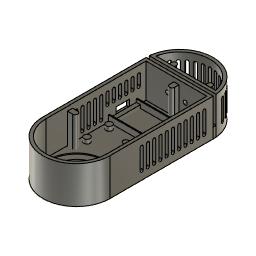
Krabicka pro termostat (Autodesk Fusion 360 design; units mm, degrees)
Autodesk Fusion 360 part; units mm, degrees
note: some values were not read from the file. Chosen so that the rebuilt part matches the saved one: which bodies a step acts on; which face or edge a step refers to. Set by a fixed rule: which sketch regions a step uses.
sketch "Sketch1" plane through (0, 0, 0) normal (0, 0, 1) x (1, 0, 0)
  circle A0 centre (0.0005, 0) radius 20.75
  arc A1 (32.4989, 100) -> (-32.5011, 100) centre (-0.0011, 100) ccw
  circle A2 centre (0.0005, 0) radius 27
  circle A3 centre (-23.4995, 33.6708) radius 3
  circle A4 centre (23.5005, 55.0015) radius 3
  circle A5 centre (23.4975, 33.1458) radius 3
  circle A6 centre (-23.4995, 55.25) radius 3
  line L0 (-26.4995, 58.5) -> (26.5005, 58.5) construction
  line L1 (26.5005, 58.5) -> (26.5005, 30) construction
  line L2 (26.5005, 30) -> (-26.4995, 30) construction
  line L3 (-26.4995, 30) -> (-26.4995, 58.5) construction
  line L4 (-49, 0) -> (63, 0)
  line L5 (-32.5011, 100) -> (32.4989, 100)
  line L6 (-32.5011, 100) -> (-32.4995, 0)
  line L7 (32.4989, 100) -> (32.5005, 0)
  arc A7 (-32.4995, 0) -> (32.5005, 0.0005) centre (0.0005, 0) ccw
  arc A8 (-29.5001, 0) -> (29.5005, 0) centre (0.0002, 0) ccw
  line L8 (-29.501, 88.5) -> (6.4991, 88.5)
  line L9 (6.4991, 88.5) -> (6.4991, 60.5)
  line L10 (6.4991, 60.5) -> (-29.5007, 60.5)
  line L11 (-29.501, 87.5) -> (5.5005, 87.5)
  line L12 (5.5005, 87.5) -> (5.5005, 61.5)
  line L13 (5.5005, 61.5) -> (-29.5007, 61.5)
  line L14 (-29.4995, 61.5) -> (-29.4995, 87.5)
  line L15 (8.7491, 92.5) -> (27.2491, 92.5) construction
  line L16 (27.2491, 92.5) -> (27.2491, 60.5) construction
  line L17 (27.2491, 60.5) -> (8.7491, 60.5) construction
  line L18 (8.7491, 60.5) -> (8.7491, 92.5) construction
  line L19 (27.2491, 74.5) -> (8.7491, 74.5)
  line L20 (27.2491, 80.5) -> (8.7491, 80.5)
  line L21 (-29.5011, 97) -> (29.4989, 97)
  line L22 (-32.3624, 103) -> (32.3601, 103)
  line L23 (-28.8845, 106) -> (28.8823, 106)
  line L24 (-6.0011, 111) -> (5.9989, 111)
  line L25 (5.9989, 111) -> (5.9989, 126)
  line L26 (5.9989, 126) -> (-6.0011, 126)
  line L27 (-6.0011, 126) -> (-6.0011, 111)
  arc A9 (-29.3482, 103) -> (-29.5011, 99.9993) centre (-0.0011, 100) ccw
  arc A10 (29.4989, 100.0007) -> (29.3459, 103) centre (-0.0011, 100) ccw
  arc A11 (28.8823, 106) -> (-28.8845, 106) centre (-0.0011, 100) ccw
  line L28 (29.4989, 100.0007) -> (29.4989, 100)
  line L29 (29.4989, 97) -> (29.5005, 0)
  line L30 (-29.5011, 97) -> (-29.5001, 0)
  line L31 (8.7491, 80.5) -> (8.7491, 74.5)
  line L32 (27.2491, 80.5) -> (27.2491, 74.5)
  line L33 (-24.4995, 23.2909) -> (-38.4097, 23.2907) construction
  line L34 (-24.4995, 20.7909) -> (-29.5003, 20.7908)
  line L35 (-24.4996, 25.7909) -> (-29.5003, 25.7908)
  arc A12 (-24.4995, 20.7909) -> (-24.4996, 25.7909) centre (-24.4995, 23.2909) ccw
  line L36 (24.4992, 20.7913) -> (29.5001, 20.7913)
  arc A13 (24.4992, 25.7913) -> (24.4992, 20.7913) centre (24.4992, 23.2913) ccw
  line L37 (24.4992, 25.7913) -> (29.5001, 25.7913)
  line L38 (-29.5011, 97) -> (-29.5001, 0)
  line L39 (-2.5011, 92.75) -> (-2.5011, 97)
  line L40 (2.4989, 92.75) -> (2.4989, 97)
  arc A14 (-2.5011, 92.75) -> (2.4989, 92.75) centre (-0.0011, 92.75) ccw
  line L41 (-26.4995, 112) -> (22.6043, 112) construction
  line L42 (-20.0011, 112) -> (-20.0011, 106)
  line L43 (-15.0011, 112) -> (-15.0011, 106)
  arc A15 (-15.0011, 112) -> (-20.0011, 112) centre (-17.5011, 112) ccw
  line L44 (14.9994, 112) -> (15, 106)
  line L45 (19.9994, 112) -> (19.9994, 106)
  arc A16 (19.9994, 112) -> (14.9994, 112) centre (17.4994, 112.0003) ccw
  line L46 (0.0002, 0) -> (0.0007, -38) construction
  line L47 (-1.7495, -20.75) -> (1.7505, -20.75)
  line L48 (-1.7495, -22.75) -> (1.7505, -22.75)
  line L49 (-1.7495, -20.75) -> (-1.7495, -22.75)
  line L50 (1.7505, -20.75) -> (1.7505, -22.75)
  line L51 (20.7505, 1.75) -> (22.7505, 1.75)
  line L52 (20.7505, -1.75) -> (22.7505, -1.75)
  line L53 (20.7505, -1.75) -> (20.7505, 1.75)
  line L54 (22.7505, -1.75) -> (22.7505, 1.75)
  line L55 (-1.7495, 20.75) -> (-1.7496, 22.75)
  line L56 (1.7505, 20.75) -> (1.7504, 22.75)
  line L57 (1.7505, 20.75) -> (-1.7495, 20.75)
  line L58 (1.7505, 22.75) -> (-1.7496, 22.75)
  line L59 (-20.7495, -1.75) -> (-22.7495, -1.75)
  line L60 (-20.7495, 1.75) -> (-22.7495, 1.75)
  line L61 (-20.7495, 1.75) -> (-20.7495, -1.75)
  line L62 (-22.7495, 1.75) -> (-22.7495, -1.75)
  line L63 (5.5005, 74.5) -> (-60, 74.5) construction
  line L64 (-25.4995, 61.5) -> (-25.4995, 87.5)
  line L65 (1.5005, 87.5) -> (1.5005, 61.5)
  dimension "d2" = 41.5
  dimension "d3" = 65
  dimension "d65" = 6
  dimension "d66" = 6
  dimension "d68" = 6
  dimension "d69" = 6
  dimension "d70" = 47
  dimension "d72" = 47
  dimension "d76" = 54
  dimension "d79" = 53
  dimension "d80" = 28.5
  dimension "d82" = 3.25
  dimension "d88" = 65
  dimension "d91" = 100
  dimension "d92" = 6
  dimension "d93" = 9
  dimension "d94" = 9
  dimension "d99" = 30
  dimension "d104" = 28
  dimension "d107" = 3
  dimension "d109" = 18.5
  dimension "d110" = 32
  dimension "d111" = 2
  dimension "d112" = 2.25
  dimension "d114" = 35
  dimension "d115" = 14
  dimension "d116" = 6
  dimension "d118" = 26
  dimension "d122" = 12
  dimension "d123" = 15
  dimension "d124" = 6
  dimension "d125" = 5
  dimension "d144" = 5
  dimension "d145" = 8
  dimension "d148" = 5
  dimension "d149" = 4.25
  dimension "d150" = 32.5
  dimension "d151" = 5
  dimension "d152" = 15
  dimension "d153" = 12
  dimension "d226" = 360
  dimension "d229" = 4
  constraint horizontal L0
  constraint vertical L1
  constraint horizontal L2
  constraint vertical L3
  constraint concentric A0 A2
  constraint horizontal L4
  constraint concentric A0 A7
  constraint coincident L4 L6.end
  constraint coincident L7.end A7
  constraint coincident L4 L7.end
  constraint coincident L7 A7.end
  constraint coincident L4 A8.start
  constraint horizontal L8
  constraint vertical L9
  constraint horizontal L10
  constraint parallel L8 L11
  constraint parallel L9 L12
  constraint parallel L10 L13
  constraint horizontal L15
  constraint vertical L16
  constraint horizontal L17
  constraint vertical L18
  constraint horizontal L19
  constraint horizontal L20
  constraint horizontal L24
  constraint vertical L25
  constraint horizontal L26
  constraint vertical L27
  constraint parallel L5 L23
  constraint concentric A1 A10
  constraint parallel L7 L28
  constraint coincident L22 A9.start
  constraint concentric A9 A10
  constraint coincident L22 A10.end
  constraint concentric A10 A11
  constraint parallel L5 L22
  constraint coincident A1 L22.end
  constraint coincident A1 L22.start
  constraint parallel L5 L21
  constraint coincident L21.end L28
  constraint coincident L5 L28.end
  constraint collinear L28 L29
  constraint coincident L30 L11.start
  constraint coincident L14.end L11
  constraint coincident L30 L13.end
  constraint coincident L14.start L13
  constraint coincident L30 L8.start
  constraint coincident L30 L10.end
  constraint perpendicular L19 L31
  constraint perpendicular L19 L32
  constraint coincident L33.start A12.centre
  constraint parallel L33 L34
  constraint coincident L30 L34.end
  constraint parallel L33 L35
  constraint coincident L30 L35.end
  constraint coincident L39.start A14
  constraint perpendicular L21 L39
  constraint perpendicular L21 L40
  constraint coincident L39 A14.start
  constraint coincident L21 L39.end
  constraint coincident L21 L40.end
  constraint perpendicular L27 L41
  constraint coincident L41 L42.start
  constraint tangent L42 A15
  constraint perpendicular L23 L42
  constraint coincident L41 L43.start
  constraint tangent L43 A15
  constraint perpendicular L23 L43
  constraint coincident L23 L42.end
  constraint coincident L23 L43.end
  constraint coincident L41 L44.start
  constraint tangent L44 A16
  constraint coincident L41 L45.start
  constraint perpendicular L23 L45
  constraint coincident L23 L45.end
  constraint coincident L23 L44.end
  constraint coincident A8.centre L46.start
  constraint tangent A0 L47
  constraint horizontal L47
  constraint parallel L47 L48
  constraint parallel L46 L50
  constraint coincident L48 L49.end
  constraint midpoint L12 L63.start
  constraint perpendicular L12 L63
  constraint parallel L12 L65
  constraint coincident L11 L65.start
  constraint coincident L13 L65.end
  measures "d2" diameter of A0
  measures "d3" diameter of A1
  measures "d65" diameter of A3
  measures "d66" diameter of A4
  measures "d68" diameter of A5
  measures "d69" diameter of A6
  measures "d70" distance of A3.centre A5.centre
  measures "d72" horizontal distance of A4.centre A6.centre
  measures "d76" diameter of A2
  measures "d79" distance of L0.start L0.end
  measures "d80" distance of L0.start L2.end
  measures "d82" vertical distance of A6.centre L0.start
  measures "d88" diameter of A7
  measures "d91" vertical distance of A1.centre A0.centre
  measures "d92" horizontal distance of L2.end L6.end
  measures "d93" horizontal distance of A3.centre L6.end
  measures "d94" horizontal distance of A6.centre L6.end
  measures "d99" vertical distance of L2.end L4.start
  measures "d104" distance of L8.end L9.end
  measures "d107" horizontal distance of L6.end L14.start
  measures "d109" distance of L15.start L15.end
  measures "d110" distance of L15.start L17.end
  measures "d111" vertical distance of L0.start L17.end
  measures "d112" distance of L9.end L17.end
  measures "d114" distance of L14.end L11.end
  measures "d115" distance of L16.end L19.start
  measures "d116" distance of L19.start L20.start
  measures "d118" distance of L14.end L14.start
  measures "d122" distance of L24.start L24.end
  measures "d123" distance of L24.start L26.end
  measures "d124" horizontal distance of A1.centre L24.end
  measures "d125" vertical distance of L24.end L23.end
  measures "d144" diameter of A12
  measures "d145" horizontal distance of L6.end L33.start
  measures "d148" diameter of A14
  measures "d149" vertical distance of L21.start A14.centre
  measures "d150" horizontal distance of A1.end A14.centre
  measures "d151" diameter of A15
  measures "d152" horizontal distance of A1.end A15.centre
  measures "d153" vertical distance of A1.end A15.centre
extrude "Extrude11" add sketch "Sketch1" along normal blind 2 contours L47 L48 L49 L50 | A0 A2 L4 L52 L53 L54 L59 L61 L62 | L4 L51 L53 L54 | L4 L52 L53 L54 | L55 L56 L57 L58 | A0 A2 L4 L51 L53 L54 L60 L61 L62 | L4 L59 L61 L62 | L4 L60 L61 L62 makes body 1
extrude "Extrude12" add sketch "Sketch1" along normal blind 3 separate body contours A2 L4 A8 | A2 L4 L8 L9 L10 L21 L29 L30 L34 L35 A12 L36 A13 L37 L38 L39 L40 A14 | L29 L36 A13 L37 | L30 L34 L35 A12 L38 | L5 L22 A9 A10 | L21 L39 L40 A14 | L11 L13 L14 L30 L38 L64 | L11 L13 L64 L65 | L11 L12 L13 L65 | L19 L20 L31 L32 | L23 A11 L42 L43 A15 L44 L45 A16 | L23 L42 L43 A15 | L23 L44 L45 A16 makes body 2 at (-9.8345, 100, 1) makes body 3 at (-5.4383, 47.1243, 0) makes body 4 at (8.7413, 120.9475, 0) makes body 5 at (-17.8337, 78.8333, 0)
extrude "Extrude13" add sketch "Sketch1" along normal blind 36 separate body contours L4 L5 L6 L7 L14 L21 L29 L30 L38 | L4 A7 A8 | A1 L22 makes body 6 at (21.5052, -24.3679, 24) makes body 7 at (-32.1753, 104.5904, 24)
extrude "Extrude14" add sketch "Sketch1" along normal blind 10 separate body contours A1 L5 L22 A10 | A1 L5 L22 A9 makes body 8 at (30.3507, 103, 3.3333) makes body 9 at (-31.3576, 103, 3.3333)
extrude "Extrude15" add sketch "Sketch1" along normal blind 7 separate body contours A3 | A4 | A5 | A6 makes body 10 at (-26.4846, 54.9513, 4.6667) makes body 11 at (20.5154, 54.7028, 4.6667) makes body 12 at (-26.4846, 33.3721, 4.6667) makes body 13 at (20.5124, 32.8471, 4.6667)
extrude "Extrude16" add sketch "Sketch1" along normal blind 9 separate body contours L8 L9 L10 L11 L12 L13 L30 L38 makes body 14
extrude "Extrude17" add sketch "Sketch1" along normal blind 8 separate body contours L24 L25 L26 L27 makes body 15
extrude "Extrude18" add sketch "Sketch1" along normal blind 7 separate body contours L19 L20 L31 L32 makes body 16
extrude "Extrude19" add sketch "Sketch1" along normal blind 32 separate body contours L29 L36 A13 L37 | L30 L34 L35 A12 L38 | L21 L39 L40 A14 | L23 L42 L43 A15 | L23 L44 L45 A16 makes body 17 at (19.9221, 112.6169, 21.3333) makes body 18 at (22.3991, 24.6477, 21.3333) makes body 19 at (-19.6343, 113.3036, 10.6667) makes body 20 at (-22.8925, 21.3758, 21.3333) makes body 21 at (2.4216, 92.1331, 21.3333)
sketch "Sketch6" plane through (0, 100, 0) normal (0, 1, 0) x (-1, 0, 0)
  line L0 (-32.4989, 0) -> (32.5011, 0)
  line L1 (32.5011, 0) -> (32.5011, 36)
  line L2 (32.5011, 36) -> (-32.4989, 36)
  line L3 (-32.4989, 36) -> (-32.4989, 0)
  line L4 (0, 0) -> (0, 60.6352)
  line L5 (-45, 18) -> (-11, 18) construction
  line L6 (0, 40) -> (0, 4) construction
  line L7 (-1.5, 18) -> (-1.5, 8)
  line L8 (1.5, 18) -> (1.5, 8)
  arc A0 (-1.5, 8) -> (1.5, 8) centre (0, 8) ccw
  arc A1 (1.5, 28) -> (-1.5, 28) centre (0, 28) ccw
  line L9 (1.5, 18) -> (1.5, 28)
  line L10 (-1.5, 18) -> (-1.5, 28)
  line L11 (32.5011, 36) -> (-32.4989, 36)
  line L12 (-32.4989, 36) -> (-32.4989, 0)
  line L13 (-32.4989, 0) -> (32.5011, 0)
  line L14 (32.5011, 0) -> (32.5011, 36)
  circle A2 centre (8.5011, 20) radius 2
  circle A3 centre (8.5011, 20) radius 3
  circle A4 centre (-8.5011, 20) radius 3
  circle A5 centre (-8.5011, 20) radius 2
  point P0 (-63, 0)
  dimension "d167" = 3
  dimension "d170" = 10
  dimension "d171" = 8
  dimension "d172" = 1.5
  dimension "d188" = 4
  dimension "d189" = 6
  dimension "d190" = 20
  dimension "d191" = 24
  constraint coincident L4.start origin
  constraint vertical L4
  constraint horizontal L5
  constraint vertical L6
  constraint coincident A0.centre L6
  constraint parallel L6 L7
  constraint parallel L6 L8
  constraint coincident L5 L7.start
  constraint coincident L5 L8.start
  constraint symmetric L5 L7.end A1.end
  constraint symmetric L5 L8.end A1.start
  constraint symmetric L5 A0 A1
  constraint symmetric L5 L7.start L10.start
  constraint symmetric L5 L8.start L9.start
  constraint horizontal L11
  constraint vertical L12
  constraint horizontal L13
  constraint vertical L14
  constraint coincident L0.start L3.end
  constraint coincident L1.end L2.start
  constraint concentric A2 A3
  constraint symmetric L4 A2 A5
  constraint symmetric L4 A3 A4
  measures "d167" diameter of A0
  measures "d170" vertical distance of A0.centre L5.start
  measures "d171" vertical distance of A0.centre P0
  measures "d172" distance of L4 L7.end
  measures "d188" diameter of A2
  measures "d189" diameter of A3
  measures "d190" vertical distance of L0.end A2.centre
  measures "d191" distance of L14 A2.centre
extrude "Extrude21" add sketch "Sketch6" along normal blind 68 separate body contours L4 L7 A0 A1 L10 | L4 L8 A0 A1 L9 makes body 22
pattern_circular "C-Pattern1" count 7 over 70 about axis through (0, 100, 0) along (0, 0, 1) of bodies 22 makes body 23 at (-7.6982, 144.7001, 21.3333) makes body 24 at (-7.6005, 121.407, 21.3333) makes body 25 at (-11.7723, 119.4278, 21.3333) makes body 26 at (-31.9449, 132.2007, 24.6667) makes body 27 at (-37.7965, 125.0756, 21.3333) makes body 28 at (-42.0864, 116.9145, 21.3333)
pattern_circular "C-Pattern2" count 7 over 70 about axis through (0, 100, 0) along (0, 0, -1) of bodies 22 makes body 29 at (10.6362, 144.0934, 21.3333) makes body 30 at (19.3329, 141.0317, 21.3333) makes body 31 at (14.2298, 117.7071, 21.3333) makes body 32 at (17.5165, 114.4638, 24.6667) makes body 33 at (39.3714, 122.5223, 21.3333) makes body 34 at (43.1124, 114.0954, 24.6667)
extrude "Extrude22" add sketch "Sketch6" along normal blind 7 separate body contours L0 L2 L3 L4 L7 A0 A1 L10 L11 L12 L13 | L0 L1 L2 L4 L8 A0 A1 L9 L11 L13 L14 | L4 L7 A0 A1 L10 | L4 L8 A0 A1 L9 | A2 | A3 | A4 | A5 makes body 35
combine "Combine1" operation cut target body 28 tool bodies 35 keep tools makes body 36 at (-1.4619, 100, 14.6667)
combine "Combine2" operation cut target body 27 tool bodies 35 keep tools makes body 37 at (-0.9524, 100, 14.6667)
combine "Combine3" operation cut target body 26 tool bodies 35 keep tools makes body 38 at (-0.7286, 100, 21.3333)
combine "Combine4" operation cut target body 25 tool bodies 35 keep tools makes body 39 at (-0.6104, 100, 21.3333)
combine "Combine5" operation cut target body 24 tool bodies 35 keep tools makes body 40 at (-0.5445, 100, 14.6667)
combine "Combine6" operation cut target body 23 tool bodies 35 keep tools makes body 41 at (-0.5105, 100, 14.6667)
combine "Combine7" operation cut target body 22 tool bodies 35 keep tools
combine "Combine8" operation cut target body 29 tool bodies 35 keep tools makes body 42 at (0.5105, 100, 21.3333)
combine "Combine9" operation cut target body 30 tool bodies 35 keep tools makes body 43 at (0.5445, 100, 21.3333)
combine "Combine10" operation cut target body 31 tool bodies 35 keep tools makes body 44 at (0.6104, 100, 21.3333)
combine "Combine11" operation cut target body 32 tool bodies 35 keep tools makes body 45 at (0.7286, 100, 21.3333)
combine "Combine12" operation cut target body 33 tool bodies 35 keep tools makes body 46 at (0.9524, 100, 21.3333)
combine "Combine13" operation cut target body 34 tool bodies 35 makes body 47 at (1.4619, 100, 21.3333)
combine "Combine14" operation cut target body 7 tool bodies 28 27 26 25 24 23 22 29 30 31 32 33 34
combine "Combine15" operation add target body 6 tool bodies 36 37 38 39 40 41 42 43 44 45 46 47
sketch "Sketch8" plane through (6.4991, 0, 0) normal (1, 0, 0) x (0, 1, 0)
  line L0 (60.5, 0) -> (88.5, 0)
  line L1 (88.5, 0) -> (88.5, 9)
  line L2 (88.5, 9) -> (60.5, 9)
  line L3 (60.5, 9) -> (60.5, 0)
  line L4 (68, 12) -> (81, 12)
  line L5 (81, 12) -> (81, 5)
  line L6 (81, 5) -> (68, 5)
  line L7 (68, 5) -> (68, 12)
  line L8 (0, 3) -> (97, 3)
  dimension "d181" = 13
  dimension "d182" = 7
  dimension "d183" = 5
  dimension "d184" = 7.5
  constraint horizontal L4
  constraint vertical L5
  constraint horizontal L6
  constraint vertical L7
  measures "d181" distance of L5.end L6.end
  measures "d182" distance of L4.end L5.end
  measures "d183" vertical distance of L0.start L6.end
  measures "d184" distance of L3 L6.end
extrude "Extrude23" add sketch "Sketch8" against normal blind 43 separate body contours L2 L4 L5 L7 | L2 L5 L6 L7 makes body 48
combine "Combine16" operation cut target body 6 tool bodies 48
extrude "Extrude24" add sketch "Sketch6" along normal blind 6 separate body contours A4 makes body 49
extrude "Extrude25" add sketch "Sketch6" along normal blind 6 separate body contours A3 makes body 50
extrude "Extrude26" add sketch "Sketch6" along normal mid plane 20 separate body contours A2 | A5 makes body 51 at (-10.4986, 106.6667, 19.9003) makes body 52 at (6.5036, 106.6667, 19.9003)
combine "Combine17" operation cut target body 6 tool bodies 51 52 keep tools
combine "Combine18" operation cut target body 7 tool bodies 51 52
sketch "Sketch10" plane through (32.5005, 0.0005, 0) normal (1, 0.000016, 0) x (-0.000016, 1, 0)
  line L0 (0, 0) -> (99.9995, 0)
  line L1 (99.9995, 0) -> (99.9995, 36)
  line L2 (99.9995, 36) -> (0, 36)
  line L3 (-13.5, 18) -> (31.5, 18) construction
  line L4 (6.5, 8) -> (6.5, 78) construction
  line L5 (32.2857, 8) -> (32.2857, 18)
  line L6 (29.2857, 8) -> (29.2857, 18)
  line L7 (29.2857, 28) -> (29.2857, 18)
  line L8 (32.2857, 28) -> (32.2857, 18)
  arc A0 (32.2857, 28) -> (29.2857, 28) centre (30.7857, 28) ccw
  arc A1 (29.2857, 8) -> (32.2857, 8) centre (30.7857, 8) ccw
  line L9 (38.3571, 8) -> (38.3571, 18)
  line L10 (35.3571, 8) -> (35.3571, 18)
  line L11 (35.3571, 28) -> (35.3571, 18)
  line L12 (38.3571, 28) -> (38.3571, 18)
  arc A2 (38.3571, 28) -> (35.3571, 28) centre (36.8571, 28) ccw
  arc A3 (35.3571, 8) -> (38.3571, 8) centre (36.8571, 8) ccw
  line L13 (44.4286, 8) -> (44.4286, 18)
  line L14 (41.4286, 8) -> (41.4286, 18)
  line L15 (41.4286, 28) -> (41.4286, 18)
  line L16 (44.4286, 28) -> (44.4286, 18)
  arc A4 (44.4286, 28) -> (41.4286, 28) centre (42.9286, 28) ccw
  arc A5 (41.4286, 8) -> (44.4286, 8) centre (42.9286, 8) ccw
  line L17 (50.5, 8) -> (50.5, 18)
  line L18 (47.5, 8) -> (47.5, 18)
  line L19 (47.5, 28) -> (47.5, 18)
  line L20 (50.5, 28) -> (50.5, 18)
  arc A6 (50.5, 28) -> (47.5, 28) centre (49, 28) ccw
  arc A7 (47.5, 8) -> (50.5, 8) centre (49, 8) ccw
  line L21 (56.5714, 8) -> (56.5714, 18)
  line L22 (53.5714, 8) -> (53.5714, 18)
  line L23 (53.5714, 28) -> (53.5714, 18)
  line L24 (56.5714, 28) -> (56.5714, 18)
  arc A8 (56.5714, 28) -> (53.5714, 28) centre (55.0714, 28) ccw
  arc A9 (53.5714, 8) -> (56.5714, 8) centre (55.0714, 8) ccw
  line L25 (62.6429, 8) -> (62.6429, 18)
  line L26 (59.6429, 8) -> (59.6429, 18)
  line L27 (59.6429, 28) -> (59.6429, 18)
  line L28 (62.6429, 28) -> (62.6429, 18)
  arc A10 (62.6429, 28) -> (59.6429, 28) centre (61.1429, 28) ccw
  arc A11 (59.6429, 8) -> (62.6429, 8) centre (61.1429, 8) ccw
  line L29 (68.7143, 8) -> (68.7143, 18)
  line L30 (65.7143, 8) -> (65.7143, 18)
  line L31 (65.7143, 28) -> (65.7143, 18)
  line L32 (68.7143, 28) -> (68.7143, 18)
  arc A12 (68.7143, 28) -> (65.7143, 28) centre (67.2143, 28) ccw
  arc A13 (65.7143, 8) -> (68.7143, 8) centre (67.2143, 8) ccw
  line L33 (74.7857, 8) -> (74.7857, 18)
  line L34 (71.7857, 8) -> (71.7857, 18)
  line L35 (71.7857, 28) -> (71.7857, 18)
  line L36 (74.7857, 28) -> (74.7857, 18)
  arc A14 (74.7857, 28) -> (71.7857, 28) centre (73.2857, 28) ccw
  arc A15 (71.7857, 8) -> (74.7857, 8) centre (73.2857, 8) ccw
  line L37 (80.8571, 8) -> (80.8571, 18)
  line L38 (77.8571, 8) -> (77.8571, 18)
  line L39 (77.8571, 28) -> (77.8571, 18)
  line L40 (80.8571, 28) -> (80.8571, 18)
  arc A16 (80.8571, 28) -> (77.8571, 28) centre (79.3571, 28) ccw
  arc A17 (77.8571, 8) -> (80.8571, 8) centre (79.3571, 8) ccw
  line L41 (86.9286, 8) -> (86.9286, 18)
  line L42 (83.9286, 8) -> (83.9286, 18)
  line L43 (83.9286, 28) -> (83.9286, 18)
  line L44 (86.9286, 28) -> (86.9286, 18)
  arc A18 (86.9286, 28) -> (83.9286, 28) centre (85.4286, 28) ccw
  arc A19 (83.9286, 8) -> (86.9286, 8) centre (85.4286, 8) ccw
  line L45 (93, 8) -> (93, 18)
  line L46 (90, 8) -> (90, 18)
  line L47 (90, 28) -> (90, 18)
  line L48 (93, 28) -> (93, 18)
  arc A20 (93, 28) -> (90, 28) centre (91.5, 28) ccw
  arc A21 (90, 8) -> (93, 8) centre (91.5, 8) ccw
  dimension "d199" = 10
  dimension "d203" = 18
  constraint horizontal L3
  measures "d199" vertical distance of L3.start L4.start
  measures "d203" vertical distance of L2.end L3.start
sketch "Sketch11" plane through (-32.4995, -0.0005, 0) normal (-1, -0.000016, 0) x (0.000016, -1, 0)
  line L0 (-81.0005, 5) -> (-81.0005, 12)
  line L1 (-81.0005, 12) -> (-68.0005, 12)
  line L2 (-68.0005, 12) -> (-68.0005, 5)
  line L3 (-68.0005, 5) -> (-81.0005, 5)
  line L4 (-100.0005, 0) -> (-0.0005, 0)
  line L5 (-0.0005, 0) -> (-0.0005, 36)
  line L6 (-0.0005, 36) -> (-100.0005, 36)
  line L7 (-100.0005, 36) -> (-100.0005, 0)
  line L8 (-22, 18) -> (11, 18) construction
  line L9 (-29.2857, 31) -> (-29.2857, 5) construction
  line L10 (-35.3571, 31) -> (-35.3571, 5) construction
  line L11 (-41.4286, 31) -> (-41.4286, 5) construction
  line L12 (-47.5, 31) -> (-47.5, 5) construction
  line L13 (-53.5714, 31) -> (-53.5714, 5) construction
  line L14 (-59.6429, 31) -> (-59.6429, 5) construction
  line L15 (-65.7143, 31) -> (-65.7143, 5) construction
  line L16 (-71.7857, 31) -> (-71.7857, 5) construction
  line L17 (-77.8571, 31) -> (-77.8571, 5) construction
  line L18 (-83.9286, 31) -> (-83.9286, 5) construction
  line L19 (-90, 31) -> (-90, 5) construction
  arc A0 (-30.7857, 8) -> (-27.7857, 8) centre (-29.2857, 8) ccw
  line L20 (-27.7857, 18) -> (-27.7857, 8)
  line L21 (-30.7857, 18) -> (-30.7857, 8)
  line L22 (-30.7857, 18) -> (-30.7857, 28)
  arc A1 (-27.7857, 28) -> (-30.7857, 28) centre (-29.2857, 28) ccw
  line L23 (-27.7857, 18) -> (-27.7857, 28)
  arc A2 (-36.8571, 8) -> (-33.8571, 8) centre (-35.3571, 8) ccw
  line L24 (-33.8571, 18) -> (-33.8571, 8)
  line L25 (-36.8571, 18) -> (-36.8571, 8)
  line L26 (-36.8571, 18) -> (-36.8571, 28)
  arc A3 (-33.8571, 28) -> (-36.8571, 28) centre (-35.3571, 28) ccw
  line L27 (-33.8571, 18) -> (-33.8571, 28)
  arc A4 (-42.9286, 8) -> (-39.9286, 8) centre (-41.4286, 8) ccw
  line L28 (-39.9286, 18) -> (-39.9286, 8)
  line L29 (-42.9286, 18) -> (-42.9286, 8)
  line L30 (-42.9286, 18) -> (-42.9286, 28)
  arc A5 (-39.9286, 28) -> (-42.9286, 28) centre (-41.4286, 28) ccw
  line L31 (-39.9286, 18) -> (-39.9286, 28)
  arc A6 (-49, 8) -> (-46, 8) centre (-47.5, 8) ccw
  line L32 (-46, 18) -> (-46, 8)
  line L33 (-49, 18) -> (-49, 8)
  line L34 (-49, 18) -> (-49, 28)
  arc A7 (-46, 28) -> (-49, 28) centre (-47.5, 28) ccw
  line L35 (-46, 18) -> (-46, 28)
  arc A8 (-55.0714, 8) -> (-52.0714, 8) centre (-53.5714, 8) ccw
  line L36 (-52.0714, 18) -> (-52.0714, 8)
  line L37 (-55.0714, 18) -> (-55.0714, 8)
  line L38 (-55.0714, 18) -> (-55.0714, 28)
  arc A9 (-52.0714, 28) -> (-55.0714, 28) centre (-53.5714, 28) ccw
  line L39 (-52.0714, 18) -> (-52.0714, 28)
  line L40 (-61.1429, 18) -> (-61.1429, 28)
  arc A10 (-58.1429, 28) -> (-61.1429, 28) centre (-59.6429, 28) ccw
  line L41 (-58.1429, 18) -> (-58.1429, 28)
  arc A11 (-61.1429, 18) -> (-58.1429, 18) centre (-59.6429, 18) ccw
  arc A12 (-64.2143, 28) -> (-67.2143, 28) centre (-65.7143, 28) ccw
  line L42 (-64.2143, 18) -> (-64.2143, 28)
  arc A13 (-67.2143, 18) -> (-64.2143, 18) centre (-65.7143, 18) ccw
  line L43 (-67.2143, 18) -> (-67.2143, 28)
  arc A14 (-70.2857, 28) -> (-73.2857, 28) centre (-71.7857, 28) ccw
  line L44 (-70.2857, 18) -> (-70.2857, 28)
  arc A15 (-73.2857, 18) -> (-70.2857, 18) centre (-71.7857, 18) ccw
  line L45 (-73.2857, 18) -> (-73.2857, 28)
  line L46 (-76.3571, 18) -> (-76.3571, 28)
  arc A16 (-76.3571, 28) -> (-79.3571, 28) centre (-77.8571, 28) ccw
  line L47 (-79.3571, 18) -> (-79.3571, 28)
  arc A17 (-79.3571, 18) -> (-76.3571, 18) centre (-77.8571, 18) ccw
  arc A18 (-82.4286, 28) -> (-85.4286, 28) centre (-83.9286, 28) ccw
  line L48 (-85.4286, 18) -> (-85.4286, 28)
  arc A19 (-85.4286, 18) -> (-82.4286, 18) centre (-83.9286, 18) ccw
  line L49 (-82.4286, 18) -> (-82.4286, 28)
  arc A20 (-88.5, 28) -> (-91.5, 28) centre (-90, 28) ccw
  line L50 (-88.5, 18) -> (-88.5, 28)
  arc A21 (-91.5, 18) -> (-88.5, 18) centre (-90, 18) ccw
  line L51 (-91.5, 18) -> (-91.5, 28)
  dimension "d213" = 18
  constraint midpoint L14 A11.centre
  constraint tangent L41 A11
  constraint tangent L42 A13
  constraint tangent L44 A15
  constraint tangent L46 A17
  constraint tangent A19 L49
  constraint tangent L50 A21
  measures "d213" vertical distance of origin L8.end
extrude "Extrude27" add sketch "Sketch1" along normal blind 4 separate body contours L47 L48 L49 L50 | L4 L51 L53 L54 | L4 L52 L53 L54 | L55 L56 L57 L58 | L4 L59 L61 L62 | L4 L60 L61 L62 makes body 53 at (0.5838, 22.75, 1.3333) makes body 54 at (22.7505, -0.5833, 1.3333) makes body 55 at (-22.7495, 0.5833, 1.3333) makes body 56 at (-0.5829, -22.75, 1.3333)
extrude "Extrude28" add sketch "Sketch1" along normal blind 6 separate body contours L11 L13 L14 L30 L38 L64 makes body 57
extrude "Extrude29" add sketch "Sketch1" along normal blind 5 separate body contours L11 L12 L13 L65 makes body 58
extrude "Extrude30" cut sketch "Sketch10" against normal blind 3 bodies 6
extrude "Extrude31" cut sketch "Sketch11" against normal blind 3 contours A0 L20 L21 L22 A1 L23 | A2 L24 L25 L26 A3 L27 | A4 L28 L29 L30 A5 L31 | A6 L32 L33 L34 A7 L35 | A8 L36 L37 L38 A9 L39 | L40 A10 L41 A11 | A12 L42 A13 L43 | A14 L44 A15 L45 | L46 A16 L47 A17 | A18 L48 A19 L49 | A20 L50 A21 L51 bodies 6
extrude "Extrude6" [suppressed]
extrude "Extrude7" [suppressed]
sketch "Sketch3" plane through (-30, 0, 0) normal (-1, 0, 0) x (0, -1, 0)
  line L0 (-60, 0) -> (0, 0)
  line L1 (0, 0) -> (0, 36)
  line L2 (0, 36) -> (-60, 36)
  line L3 (-60, 36) -> (-60, 0)
  line L4 (-52, 8) -> (-52, 28)
  line L5 (-55, 28) -> (-55, 8)
  arc A0 (-52, 28) -> (-55, 28) centre (-53.5, 28) ccw
  arc A1 (-55, 8) -> (-52, 8) centre (-53.5, 8) ccw
  arc A2 (-46.125, 28) -> (-49.125, 28) centre (-47.625, 28) ccw
  line L6 (-46.125, 8) -> (-46.125, 28)
  line L7 (-49.125, 28) -> (-49.125, 8)
  arc A3 (-49.125, 8) -> (-46.125, 8) centre (-47.625, 8) ccw
  arc A4 (-40.25, 28) -> (-43.25, 28) centre (-41.75, 28) ccw
  line L8 (-40.25, 8) -> (-40.25, 28)
  line L9 (-43.25, 28) -> (-43.25, 8)
  arc A5 (-43.25, 8) -> (-40.25, 8) centre (-41.75, 8) ccw
  arc A6 (-34.375, 28) -> (-37.375, 28) centre (-35.875, 28) ccw
  line L10 (-34.375, 8) -> (-34.375, 28)
  line L11 (-37.375, 28) -> (-37.375, 8)
  arc A7 (-37.375, 8) -> (-34.375, 8) centre (-35.875, 8) ccw
  arc A8 (-28.5, 28) -> (-31.5, 28) centre (-30, 28) ccw
  line L12 (-28.5, 8) -> (-28.5, 28)
  line L13 (-31.5, 28) -> (-31.5, 8)
  arc A9 (-31.5, 8) -> (-28.5, 8) centre (-30, 8) ccw
  arc A10 (-22.625, 28) -> (-25.625, 28) centre (-24.125, 28) ccw
  line L14 (-22.625, 8) -> (-22.625, 28)
  line L15 (-25.625, 28) -> (-25.625, 8)
  arc A11 (-25.625, 8) -> (-22.625, 8) centre (-24.125, 8) ccw
  arc A12 (-16.75, 28) -> (-19.75, 28) centre (-18.25, 28) ccw
  line L16 (-16.75, 8) -> (-16.75, 28)
  line L17 (-19.75, 28) -> (-19.75, 8)
  arc A13 (-19.75, 8) -> (-16.75, 8) centre (-18.25, 8) ccw
  arc A14 (-10.875, 28) -> (-13.875, 28) centre (-12.375, 28) ccw
  line L18 (-10.875, 8) -> (-10.875, 28)
  line L19 (-13.875, 28) -> (-13.875, 8)
  arc A15 (-13.875, 8) -> (-10.875, 8) centre (-12.375, 8) ccw
  arc A16 (-5, 28) -> (-8, 28) centre (-6.5, 28) ccw
  line L20 (-5, 8) -> (-5, 28)
  line L21 (-8, 28) -> (-8, 8)
  arc A17 (-8, 8) -> (-5, 8) centre (-6.5, 8) ccw
  line L22 (-60, 18) -> (-55, 18)
  dimension "d42" = 3
  dimension "d43" = 20
  dimension "d44" = 3
  dimension "d45" = 3
  dimension "d46" = 10
  dimension "d47" = 5
  dimension "d50" = 47
  dimension "d51" = 0
  constraint vertical L4
  constraint vertical L5
  constraint midpoint L3 L22.start
  constraint coincident L5 L22.end
  measures "d42" distance of L5.end L4.start
  measures "d43" distance of L5.end L5.start
  measures "d44" diameter of A1
  measures "d45" diameter of A0
  measures "d46" vertical distance of A0.centre L22.start
  measures "d47" horizontal distance of L5.end L22.start
extrude "Extrude8" [suppressed]
extrude "Extrude9" [suppressed]
named bodies: "Prstenec pro zásuvku", "Dělící mezera", "Hlavní tělo", "Prostor pro čidlo", "Prostor pod čipem", "Hlavní prostor", "Prostor s čidlem", "Pravý spoj", "Levý spoj", "Rele - 1", "Rele - 2", "Rele - 3", "Rele - 4", "Ohradka na čip", "Čidlo", "Pod trafo", "Šroub - čidlo - 1", "Šroub - Hlavní - 1", "Šroub - čidlo - 2", "Šroub - Hlavní - 2", "Šroub - Hlavní - 3"
